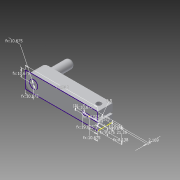
# Autodesk Inventor part: Egg_Turner_Motor_Arm
Saved by Autodesk Inventor 2014 (Build 180170000, 170)
## iProperties
Created: 2014-06-07
Part Number: Egg_Turner_Motor_Arm
Material: Generic
Document SubType Name: Modeling
Designer: mattsc
Density: 1 g/cm^3
Appearance: Default
Author: mattsc
Autodesk Inventor part; units mm, degrees
ref_plane "YZ Plane" through (0, 0, 0) normal (1, 0, 0) x (0, 1, 0)
ref_plane "XZ Plane" through (0, 0, 0) normal (0, 1, 0) x (-1, 0, 0)
ref_plane "XY Plane" through (0, 0, 0) normal (0, 0, 1) x (1, 0, 0)
sketch "Bottom" plane through (0, 0, 0) normal (0, 1, 0) x (-1, 0, 0)
  line L0 (-10.675, -10.675) -> (82.525, -10.675)
  line L1 (82.525, -10.675) -> (82.525, 10.675)
  line L2 (82.525, 10.675) -> (-10.675, 10.675)
  line L3 (-10.675, 10.675) -> (-10.675, -10.675) construction
  line L4 (-10.675, 1.5) -> (8.35, 1.5)
  line L5 (8.35, 1.5) -> (8.35, -1.5)
  line L6 (8.35, -1.5) -> (-10.675, -1.5)
  line L7 (-10.675, 1.5) -> (-10.675, 10.675)
  line L8 (-10.675, -1.5) -> (-10.675, -10.675)
  circle A0 centre (71.85, 0) radius 5.3375
  point P0 (0, 0)
  point P1 (8.35, 0)
  dimension "Width" = 21.35
  dimension "d2" = 10.675
  dimension "d3" = 93.2
  dimension "d4" = 10.675
  dimension "d8" = 9.175
  dimension "d9" = 9.175
  dimension "d10" = 3
  dimension "ArmMount" = 19.025
  dimension "d15" = 19.025
  dimension "d16" = 10.675
  dimension "d19" = 10.675
  dimension "d22" = 10.675
  dimension "d23" = 10.675
  constraints: 18 end point, 3 parallel, 2 collinear, 2 horizontal, 2 perpendicular, 1 centre point, 1 point on line
  measures "Width" distance between parallel lines of L0 L2
  measures "d2" distance from line of L2 point (0, 0)
  measures "d3" distance between parallel lines of L1 L3
  measures "d4" distance from line of L3 point (0, 0)
  measures "d8" distance of L4.start L2.end
  measures "d9" distance between parallel lines of L0 L6
  measures "d10" distance of L4.end L5.end
  measures "ArmMount" distance between parallel lines of L5 L8
  measures "d15" distance from line of L3 point (8.35, 0)
  measures "d16" distance from line of L2 point (8.35, 0)
  measures "d19" diameter of A0
  measures "d22" distance from line of L2 A0.centre
  measures "d23" distance from line of L1 A0.centre
extrude "Extrusion1" add sketch "Bottom" along normal blind 19.35 contours L8 L6 L5 L4 L7 L2 L1 L0 | A0
extrude "Extrusion2" add sketch "Bottom" along normal blind 48.375 contours A0
hole "Hole1" at (-8.35, 0, 0) direction (0, 1, 0) diameter 5.5 end through all
sketch "Side" plane through (10.675, 0, -10.675) normal (0, 0, -1) x (-1, 0, 0)
  line L0 (0, 19.35) -> (93.2, 19.35) projected
  line L1 (0, 0) -> (0, 19.35) projected
  line L2 (8.1375, 2.1694) -> (1.6375, 5.9222)
  line L3 (1.6375, 5.9222) -> (1.6375, 13.4278)
  line L4 (1.6375, 13.4278) -> (8.1375, 17.1806)
  line L5 (8.1375, 17.1806) -> (14.6375, 13.4278)
  line L6 (14.6375, 13.4278) -> (14.6375, 5.9222)
  line L7 (14.6375, 5.9222) -> (8.1375, 2.1694)
  point P0 (10.675, 0)
  point P1 (8.1375, 9.675)
  point P2 (8.1375, 9.675)
  dimension "d31" = 9.675
  dimension "d32" = 8.1375
  dimension "Nut" = 6.5
  dimension "d44" = 2.1694
  constraints: 12 end point, 1 coincident, 13 other
  measures "d31" distance from line of L0 point (8.137, 9.675)
  measures "d32" distance from line of L1 point (8.137, 9.675)
  measures "Nut" distance from line of L5 point (8.137, 9.675)
  measures "d44" distance from line of L0 L4.end
hole "Hole2" at (2.5375, 9.675, -10.675) direction (0, 0, 1) diameter 6.35 end through all
extrude "Extrusion3" cut sketch "Side" against normal blind 4.5875
fillet "Fillet1" radius 10.675 2 edges at (-82.525, 9.675, -10.675) (-82.525, 9.675, 10.675)
fillet "Fillet2" radius 4 1 edges at (-66.5125, 48.375, 0)
fillet "Fillet3" radius 4.8 1 edges at (-66.5125, 19.35, 0)
equation "\"d2\" = 0.5 * Width"
equation "\"d4\" = d2"
equation "\"d9\" = d8"
equation "\"d15\" = ArmMount"
equation "\"d16\" = d2"
equation "\"d19\" = d2"
equation "\"d22\" = d2"
equation "\"d23\" = d2"
equation "\"d20\" = 2.5 * Thickness"
equation "\"d31\" = 0.5 * Thickness"
equation "\"d32\" = -0.25 * GearDiameter + 0.5 * ArmMount"
equation "\"d45\" = 0.5 * d9"
equation "\"d47\" = 0.5 * Width"
equation "\"Thickness\" = 19.35"
equation "\"GearDiameter\" = 5.5"
body "Solid1"
